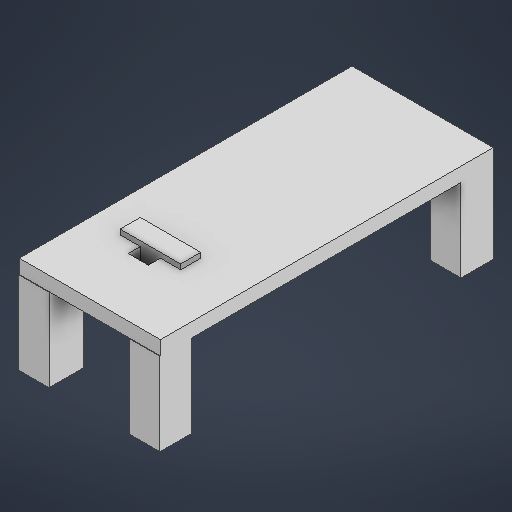
# Autodesk Inventor part: piano laterale
Saved by Autodesk Inventor 2026.2 (Build 302298000, 298)
## iProperties
Created: 2026-01-19
Part Number: piano laterale
Material: Generic
Document SubType Name: Modeling
Designer: ASUS
Density: 1 g/cm^3
Appearance: Default
Author: ASUS
Autodesk Inventor part; units mm, degrees
ref_plane "YZ Plane" through (0, 0, 0) normal (1, 0, 0) x (0, 1, 0)
ref_plane "XZ Plane" through (0, 0, 0) normal (0, 1, 0) x (-1, 0, 0)
ref_plane "XY Plane" through (0, 0, 0) normal (0, 0, 1) x (1, 0, 0)
sketch "Sketch1" plane through (0, 0, 0) normal (0, 1, 0) x (-1, 0, 0)
  line L0 (0, 0) -> (-70, 0)
  line L1 (-70, 0) -> (-70, 165)
  line L2 (-70, 165) -> (0, 165)
  line L3 (0, 165) -> (0, 0)
  dimension "d0" = 70
  dimension "d1" = 165
  constraints: 8 end point, 2 parallel, 1 horizontal, 1 perpendicular
  measures "d0" distance of L1.end L2.end
  measures "d1" distance of L0.end L1.end
extrude "Extrusion1" add sketch "Sketch1" along normal blind 7
sketch "Sketch2" plane through (0, 0, 0) normal (0, -1, 0) x (1, 0, 0)
  line L0 (70, 165) -> (70, 0) projected
  line L1 (70, 0) -> (55, 0)
  line L2 (55, 0) -> (55, 15.9792)
  line L3 (55, 15.9792) -> (70, 15.9792)
  line L4 (70, 15.9792) -> (70, 0)
  line L5 (70, 0) -> (0, 0) projected
  line L6 (0, 0) -> (15, 0)
  line L7 (15, 0) -> (15, 13.5714)
  line L8 (15, 13.5714) -> (0, 13.5714)
  line L9 (0, 13.5714) -> (0, 0)
  line L10 (70, 165.2646) -> (55, 165.2646)
  line L11 (55, 165.2646) -> (55, 149.7232)
  line L12 (55, 149.7232) -> (70, 149.7232)
  line L13 (70, 149.7232) -> (70, 165.2646)
  line L14 (0, 165.2646) -> (15, 165.2646)
  line L15 (15, 165.2646) -> (15, 148.1909)
  line L16 (15, 148.1909) -> (0, 148.1909)
  line L17 (0, 148.1909) -> (0, 165.2646)
  line L18 (68, 151.7232) -> (57, 151.7232)
  line L19 (57, 151.7232) -> (57, 163.2646)
  line L20 (57, 163.2646) -> (68, 163.2646)
  line L21 (68, 163.2646) -> (68, 151.7232)
  line L22 (2, 150.1909) -> (13, 150.1909)
  line L23 (13, 150.1909) -> (13, 163.2646)
  line L24 (13, 163.2646) -> (2, 163.2646)
  line L25 (2, 163.2646) -> (2, 150.1909)
  line L26 (2, 11.5714) -> (13, 11.5714)
  line L27 (13, 11.5714) -> (13, 2)
  line L28 (13, 2) -> (2, 2)
  line L29 (2, 2) -> (2, 11.5714)
  line L30 (68, 13.9792) -> (57, 13.9792)
  line L31 (57, 13.9792) -> (57, 2)
  line L32 (57, 2) -> (68, 2)
  line L33 (68, 2) -> (68, 13.9792)
  dimension "d4" = 15
  dimension "d5" = 15
  dimension "d6" = 15
  dimension "d7" = 15
  dimension "d8" = 2
  dimension "d9" = 2
  dimension "d10" = 2
  dimension "d11" = 2
  constraints: 64 end point, 16 parallel, 8 perpendicular, 4 horizontal, 3 point on line, 12 other
  measures "d4" distance of L2.end L3.end
  measures "d5" distance of L8.end L7.end
  measures "d6" distance of L12.end L11.end
  measures "d7" distance of L15.end L16.end
  measures "d8" distance between parallel lines of L12 L18
  measures "d9" distance between parallel lines of L16 L22
  measures "d10" distance between parallel lines of L8 L26
  measures "d11" distance between parallel lines of L3 L30
extrude "Extrusion2" add sketch "Sketch2" along normal blind 41
sketch "Sketch8" plane through (0, 7, 0) normal (0, 1, 0) x (1, 0, 0)
  line L0 (0, 0) -> (0, -165) projected
  line L1 (0, -165) -> (0, -130)
  line L2 (35, -130) -> (25, -130)
  line L3 (25, -130) -> (25, -136)
  line L4 (25, -136) -> (35, -136)
  line L5 (35, -136) -> (35, -130)
  line L6 (15, -130) -> (15, -120)
  line L7 (15, -120) -> (45, -120)
  line L8 (45, -120) -> (45, -130)
  line L9 (45, -130) -> (15, -130)
  line L10 (15, -130) -> (15, -120)
  dimension "d45" = 35
  dimension "d47" = 10
  dimension "d53" = 30
  constraints: 20 end point, 4 parallel, 2 horizontal, 2 perpendicular, 1 point on line
  measures "d45" distance of L0.end L1.end
  measures "d47" distance of L4.end L3.end
  measures "d53" distance of L8.end L9.end
extrude "Extrusion8" add sketch "Sketch8" along normal blind 2.5 contours L2 L9 L6 L7 L8
extrude "Extrusion9" cut sketch "Sketch8" against normal blind 7 contours L5 L4 L3 L2
body "Solid1"
